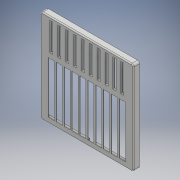
# Autodesk Inventor part: cover
Saved by Autodesk Inventor 2017 (Build 210142000, 142)
## iProperties
Created: 2017-08-24
Part Number: cover
Material: Generic
Document SubType Name: Modeling
Designer: erwin
Density: 1 g/cm^3
Appearance: Default
Author: erwin
Autodesk Inventor part; units mm, degrees
ref_plane "YZ Plane" through (0, 0, 0) normal (1, 0, 0) x (0, 1, 0)
ref_plane "XZ Plane" through (0, 0, 0) normal (0, 1, 0) x (-1, 0, 0)
ref_plane "XY Plane" through (0, 0, 0) normal (0, 0, 1) x (1, 0, 0)
sketch "Sketch1" plane through (0, 0, 0) normal (0, 1, 0) x (-1, 0, 0)
  line L0 (-45, 45) -> (45, 45)
  line L1 (45, 45) -> (45, -45)
  line L2 (45, -45) -> (-45, -45)
  line L3 (-45, -45) -> (-45, 45)
  line L4 (-45, 45) -> (45, -45) construction
  line L5 (45, 45) -> (-45, -45) construction
  line L6 (35.79, 42) -> (32.79, 42)
  line L7 (32.79, 42) -> (32.79, 15)
  line L8 (32.79, 15) -> (35.79, 15)
  line L9 (35.79, 15) -> (35.79, 42)
  line L10 (35.79, 42) -> (32.79, 15) construction
  line L11 (32.79, 42) -> (35.79, 15) construction
  line L12 (28.17, 42) -> (25.17, 42)
  line L13 (25.17, 42) -> (25.17, 15)
  line L14 (25.17, 15) -> (28.17, 15)
  line L15 (28.17, 15) -> (28.17, 42)
  line L16 (28.17, 42) -> (25.17, 15) construction
  line L17 (25.17, 42) -> (28.17, 15) construction
  line L18 (20.55, 42) -> (17.55, 42)
  line L19 (17.55, 42) -> (17.55, 15)
  line L20 (17.55, 15) -> (20.55, 15)
  line L21 (20.55, 15) -> (20.55, 42)
  line L22 (20.55, 42) -> (17.55, 15) construction
  line L23 (17.55, 42) -> (20.55, 15) construction
  line L24 (12.93, 42) -> (9.93, 42)
  line L25 (9.93, 42) -> (9.93, 15)
  line L26 (9.93, 15) -> (12.93, 15)
  line L27 (12.93, 15) -> (12.93, 42)
  line L28 (12.93, 42) -> (9.93, 15) construction
  line L29 (9.93, 42) -> (12.93, 15) construction
  line L30 (5.31, 42) -> (2.31, 42)
  line L31 (2.31, 42) -> (2.31, 15)
  line L32 (2.31, 15) -> (5.31, 15)
  line L33 (5.31, 15) -> (5.31, 42)
  line L34 (5.31, 42) -> (2.31, 15) construction
  line L35 (2.31, 42) -> (5.31, 15) construction
  line L36 (-2.31, 42) -> (-5.31, 42)
  line L37 (-5.31, 42) -> (-5.31, 15)
  line L38 (-5.31, 15) -> (-2.31, 15)
  line L39 (-2.31, 15) -> (-2.31, 42)
  line L40 (-2.31, 42) -> (-5.31, 15) construction
  line L41 (-5.31, 42) -> (-2.31, 15) construction
  line L42 (-9.93, 42) -> (-12.93, 42)
  line L43 (-12.93, 42) -> (-12.93, 15)
  line L44 (-12.93, 15) -> (-9.93, 15)
  line L45 (-9.93, 15) -> (-9.93, 42)
  line L46 (-9.93, 42) -> (-12.93, 15) construction
  line L47 (-12.93, 42) -> (-9.93, 15) construction
  line L48 (-17.55, 42) -> (-20.55, 42)
  line L49 (-20.55, 42) -> (-20.55, 15)
  line L50 (-20.55, 15) -> (-17.55, 15)
  line L51 (-17.55, 15) -> (-17.55, 42)
  line L52 (-17.55, 42) -> (-20.55, 15) construction
  line L53 (-20.55, 42) -> (-17.55, 15) construction
  line L54 (-25.17, 42) -> (-28.17, 42)
  line L55 (-28.17, 42) -> (-28.17, 15)
  line L56 (-28.17, 15) -> (-25.17, 15)
  line L57 (-25.17, 15) -> (-25.17, 42)
  line L58 (-25.17, 42) -> (-28.17, 15) construction
  line L59 (-28.17, 42) -> (-25.17, 15) construction
  line L60 (-32.79, 42) -> (-35.79, 42)
  line L61 (-35.79, 42) -> (-35.79, 15)
  line L62 (-35.79, 15) -> (-32.79, 15)
  line L63 (-32.79, 15) -> (-32.79, 42)
  line L64 (-32.79, 42) -> (-35.79, 15) construction
  line L65 (-35.79, 42) -> (-32.79, 15) construction
  line L66 (-35.79, 15) -> (35.79, 15) construction
  line L67 (35.79, 15) -> (35.79, 42) construction
  line L68 (35.79, 42) -> (-35.79, 42) construction
  line L69 (-35.79, 42) -> (-35.79, 15) construction
  line L70 (0, 42) -> (0, 45) construction
  line L71 (0, 42) -> (3, 42) construction
  line L72 (34.3728, 15) -> (34.3728, -45) construction
  line L73 (37.3728, 10) -> (31.3728, 10)
  line L74 (31.3728, 10) -> (31.3728, -40)
  line L75 (31.3728, -40) -> (37.3728, -40)
  line L76 (37.3728, -40) -> (37.3728, 10)
  line L77 (37.3728, 10) -> (31.3728, -40) construction
  line L78 (31.3728, 10) -> (37.3728, -40) construction
  line L79 (-52.62, 45) -> (37.38, -45) construction
  line L80 (23.7528, 10) -> (23.7528, -40)
  line L81 (23.7528, -40) -> (29.7528, -40)
  line L82 (29.7528, -40) -> (29.7528, 10)
  line L83 (29.7528, 10) -> (23.7528, -40) construction
  line L84 (23.7528, 10) -> (29.7528, -40) construction
  line L85 (29.7528, 10) -> (23.7528, 10)
  line L86 (-60.24, 45) -> (29.76, -45) construction
  line L87 (16.1328, 10) -> (16.1328, -40)
  line L88 (16.1328, -40) -> (22.1328, -40)
  line L89 (22.1328, -40) -> (22.1328, 10)
  line L90 (22.1328, 10) -> (16.1328, -40) construction
  line L91 (16.1328, 10) -> (22.1328, -40) construction
  line L92 (22.1328, 10) -> (16.1328, 10)
  line L93 (-67.86, 45) -> (22.14, -45) construction
  line L94 (8.5128, 10) -> (8.5128, -40)
  line L95 (8.5128, -40) -> (14.5128, -40)
  line L96 (14.5128, -40) -> (14.5128, 10)
  line L97 (14.5128, 10) -> (8.5128, -40) construction
  line L98 (8.5128, 10) -> (14.5128, -40) construction
  line L99 (14.5128, 10) -> (8.5128, 10)
  line L100 (-75.48, 45) -> (14.52, -45) construction
  line L101 (0.8928, 10) -> (0.8928, -40)
  line L102 (0.8928, -40) -> (6.8928, -40)
  line L103 (6.8928, -40) -> (6.8928, 10)
  line L104 (6.8928, 10) -> (0.8928, -40) construction
  line L105 (0.8928, 10) -> (6.8928, -40) construction
  line L106 (6.8928, 10) -> (0.8928, 10)
  line L107 (-83.1, 45) -> (6.9, -45) construction
  line L108 (-6.7272, 10) -> (-6.7272, -40)
  line L109 (-6.7272, -40) -> (-0.7272, -40)
  line L110 (-0.7272, -40) -> (-0.7272, 10)
  line L111 (-0.7272, 10) -> (-6.7272, -40) construction
  line L112 (-6.7272, 10) -> (-0.7272, -40) construction
  line L113 (-0.7272, 10) -> (-6.7272, 10)
  line L114 (-90.72, 45) -> (-0.72, -45) construction
  line L115 (-14.3472, 10) -> (-14.3472, -40)
  line L116 (-14.3472, -40) -> (-8.3472, -40)
  line L117 (-8.3472, -40) -> (-8.3472, 10)
  line L118 (-8.3472, 10) -> (-14.3472, -40) construction
  line L119 (-14.3472, 10) -> (-8.3472, -40) construction
  line L120 (-8.3472, 10) -> (-14.3472, 10)
  line L121 (-98.34, 45) -> (-8.34, -45) construction
  line L122 (-21.9672, 10) -> (-21.9672, -40)
  line L123 (-21.9672, -40) -> (-15.9672, -40)
  line L124 (-15.9672, -40) -> (-15.9672, 10)
  line L125 (-15.9672, 10) -> (-21.9672, -40) construction
  line L126 (-21.9672, 10) -> (-15.9672, -40) construction
  line L127 (-15.9672, 10) -> (-21.9672, 10)
  line L128 (-105.96, 45) -> (-15.96, -45) construction
  line L129 (-29.5872, 10) -> (-29.5872, -40)
  line L130 (-29.5872, -40) -> (-23.5872, -40)
  line L131 (-23.5872, -40) -> (-23.5872, 10)
  line L132 (-23.5872, 10) -> (-29.5872, -40) construction
  line L133 (-29.5872, 10) -> (-23.5872, -40) construction
  line L134 (-23.5872, 10) -> (-29.5872, 10)
  line L135 (-113.58, 45) -> (-23.58, -45) construction
  line L136 (-37.2072, 10) -> (-37.2072, -40)
  line L137 (-37.2072, -40) -> (-31.2072, -40)
  line L138 (-31.2072, -40) -> (-31.2072, 10)
  line L139 (-31.2072, 10) -> (-37.2072, -40) construction
  line L140 (-37.2072, 10) -> (-31.2072, -40) construction
  line L141 (-31.2072, 10) -> (-37.2072, 10)
  point P0 (0, 0)
  point P1 (34.29, 28.5)
  point P2 (26.67, 28.5)
  point P3 (19.05, 28.5)
  point P4 (11.43, 28.5)
  point P5 (3.81, 28.5)
  point P6 (-3.81, 28.5)
  point P7 (-11.43, 28.5)
  point P8 (-19.05, 28.5)
  point P9 (-26.67, 28.5)
  point P10 (-34.29, 28.5)
  point P11 (0, 45)
  point P12 (34.3728, -15)
  point P13 (26.7528, -15)
  point P14 (19.1328, -15)
  point P15 (11.5128, -15)
  point P16 (3.8928, -15)
  point P17 (-3.7272, -15)
  point P18 (-11.3472, -15)
  point P19 (-18.9672, -15)
  point P20 (-26.5872, -15)
  point P21 (-34.2072, -15)
  dimension "d0" = 90
  dimension "d1" = 90
  dimension "d2" = 3
  dimension "d3" = 27
  dimension "d6" = 7.62
  dimension "d11" = 3
  dimension "d12" = 90
  dimension "d13" = 6
  dimension "d14" = 50
  dimension "d17" = 7.62
  constraints: 284 end point, 45 midpoint, 8 parallel, 7 horizontal, 6 perpendicular, 2 collinear, 2 point on line, 1 vertical, 223 other
  measures "d0" distance of L1.end L2.end
  measures "d1" distance of L0.end L1.end
  measures "d2" distance of L8.end L7.end
  measures "d3" distance of L7.end L6.end
  measures "d6" distance of L6.start L12.start
  measures "d11" distance of L70.start L70.end
  measures "d12" angle of L71 L70
  measures "d13" distance of L75.end L74.end
  measures "d14" distance of L74.end L73.end
  measures "d17" distance of L0.start L79.start
extrude "Extrusion1" add sketch "Sketch1" along normal blind 0.5
sketch "Sketch2" plane through (0, 0.5, 0) normal (0, 1, 0) x (1, 0, 0)
  line L0 (31.2072, -10) -> (31.2072, 40)
  line L1 (31.2072, 40) -> (37.2072, 40)
  line L2 (37.2072, 40) -> (37.2072, -10)
  line L3 (37.2072, -10) -> (31.2072, -10)
  line L4 (23.5872, -10) -> (23.5872, 40)
  line L5 (23.5872, 40) -> (29.5872, 40)
  line L6 (29.5872, 40) -> (29.5872, -10)
  line L7 (29.5872, -10) -> (23.5872, -10)
  line L8 (15.9672, -10) -> (15.9672, 40)
  line L9 (15.9672, 40) -> (21.9672, 40)
  line L10 (21.9672, 40) -> (21.9672, -10)
  line L11 (21.9672, -10) -> (15.9672, -10)
  line L12 (8.3472, -10) -> (8.3472, 40)
  line L13 (8.3472, 40) -> (14.3472, 40)
  line L14 (14.3472, 40) -> (14.3472, -10)
  line L15 (14.3472, -10) -> (8.3472, -10)
  line L16 (0.7272, -10) -> (0.7272, 40)
  line L17 (0.7272, 40) -> (6.7272, 40)
  line L18 (6.7272, 40) -> (6.7272, -10)
  line L19 (6.7272, -10) -> (0.7272, -10)
  line L20 (-6.8928, -10) -> (-6.8928, 40)
  line L21 (-6.8928, 40) -> (-0.8928, 40)
  line L22 (-0.8928, 40) -> (-0.8928, -10)
  line L23 (-0.8928, -10) -> (-6.8928, -10)
  line L24 (-14.5128, -10) -> (-14.5128, 40)
  line L25 (-14.5128, 40) -> (-8.5128, 40)
  line L26 (-8.5128, 40) -> (-8.5128, -10)
  line L27 (-8.5128, -10) -> (-14.5128, -10)
  line L28 (-22.1328, -10) -> (-22.1328, 40)
  line L29 (-22.1328, 40) -> (-16.1328, 40)
  line L30 (-16.1328, 40) -> (-16.1328, -10)
  line L31 (-16.1328, -10) -> (-22.1328, -10)
  line L32 (-29.7528, -10) -> (-29.7528, 40)
  line L33 (-29.7528, 40) -> (-23.7528, 40)
  line L34 (-23.7528, 40) -> (-23.7528, -10)
  line L35 (-23.7528, -10) -> (-29.7528, -10)
  line L36 (-37.3728, -10) -> (-37.3728, 40)
  line L37 (-37.3728, 40) -> (-31.3728, 40)
  line L38 (-31.3728, 40) -> (-31.3728, -10)
  line L39 (-31.3728, -10) -> (-37.3728, -10)
  line L40 (32.79, -42) -> (32.79, -15) projected
  line L41 (32.79, -15) -> (35.79, -15) projected
  line L42 (35.79, -15) -> (35.79, -42) projected
  line L43 (35.79, -42) -> (32.79, -42) projected
  line L44 (25.17, -42) -> (25.17, -15) projected
  line L45 (25.17, -15) -> (28.17, -15) projected
  line L46 (28.17, -15) -> (28.17, -42) projected
  line L47 (28.17, -42) -> (25.17, -42) projected
  line L48 (17.55, -42) -> (17.55, -15) projected
  line L49 (17.55, -15) -> (20.55, -15) projected
  line L50 (20.55, -15) -> (20.55, -42) projected
  line L51 (20.55, -42) -> (17.55, -42) projected
  line L52 (9.93, -42) -> (9.93, -15) projected
  line L53 (9.93, -15) -> (12.93, -15) projected
  line L54 (12.93, -15) -> (12.93, -42) projected
  line L55 (12.93, -42) -> (9.93, -42) projected
  line L56 (2.31, -42) -> (2.31, -15) projected
  line L57 (2.31, -15) -> (5.31, -15) projected
  line L58 (5.31, -15) -> (5.31, -42) projected
  line L59 (5.31, -42) -> (2.31, -42) projected
  line L60 (-5.31, -42) -> (-5.31, -15) projected
  line L61 (-5.31, -15) -> (-2.31, -15) projected
  line L62 (-2.31, -15) -> (-2.31, -42) projected
  line L63 (-2.31, -42) -> (-5.31, -42) projected
  line L64 (-12.93, -42) -> (-12.93, -15) projected
  line L65 (-12.93, -15) -> (-9.93, -15) projected
  line L66 (-9.93, -15) -> (-9.93, -42) projected
  line L67 (-9.93, -42) -> (-12.93, -42) projected
  line L68 (-20.55, -42) -> (-20.55, -15) projected
  line L69 (-20.55, -15) -> (-17.55, -15) projected
  line L70 (-17.55, -15) -> (-17.55, -42) projected
  line L71 (-17.55, -42) -> (-20.55, -42) projected
  line L72 (-28.17, -42) -> (-28.17, -15) projected
  line L73 (-28.17, -15) -> (-25.17, -15) projected
  line L74 (-25.17, -15) -> (-25.17, -42) projected
  line L75 (-25.17, -42) -> (-28.17, -42) projected
  line L76 (-35.79, -42) -> (-35.79, -15) projected
  line L77 (-35.79, -15) -> (-32.79, -15) projected
  line L78 (-32.79, -15) -> (-32.79, -42) projected
  line L79 (-32.79, -42) -> (-35.79, -42) projected
  line L80 (-45, -45) -> (45, -45) projected
  line L81 (45, -45) -> (45, 45) projected
  line L82 (45, 45) -> (-45, 45) projected
  line L83 (-45, 45) -> (-45, -45) projected
  line L84 (37.2072, -10) -> (-37.3728, -10)
  line L85 (-37.3728, -10) -> (-37.3728, 40)
  line L86 (-37.3728, 40) -> (37.2072, 40)
  line L87 (37.2072, 40) -> (37.2072, -10)
  line L88 (-43.396, -12.9864) -> (42.604, -12.9864)
  line L89 (42.604, -12.9864) -> (42.604, 43.0136)
  line L90 (42.604, 43.0136) -> (-43.396, 43.0136)
  line L91 (-43.396, 43.0136) -> (-43.396, -12.9864)
  line L92 (-0.396, 43.0136) -> (-0.396, -106.8962) construction
  line L93 (-0.396, 43.0136) -> (149.5138, 43.0136) construction
  point P0 (0, 0)
  dimension "d24" = 56
  dimension "d25" = 86
  dimension "d26" = 90
  constraints: 100 end point, 4 perpendicular, 1 horizontal, 1 midpoint, 1 other
  measures "d24" distance of L88.end L89.end
  measures "d25" distance of L89.end L90.end
  measures "d26" angle of L92 L93
extrude "Extrusion2" add sketch "Sketch2" along normal blind 1.5 contours L83 L82 L81 L80
sketch "Sketch3" plane through (0, 2, 0) normal (0, 1, 0) x (1, 0, 0)
  line L0 (-43.396, -12.9864) -> (-43.396, 43.0136) projected
  line L1 (-43.396, 43.0136) -> (42.604, 43.0136) projected
  line L2 (42.604, 43.0136) -> (42.604, -12.9864) projected
  line L3 (42.604, -12.9864) -> (-43.396, -12.9864) projected
  line L4 (-35.79, -15) -> (-32.79, -15) projected
  line L5 (-32.79, -15) -> (-32.79, -42) projected
  line L6 (-32.79, -42) -> (-35.79, -42) projected
  line L7 (-35.79, -42) -> (-35.79, -15) projected
  line L8 (-28.17, -15) -> (-25.17, -15) projected
  line L9 (-25.17, -15) -> (-25.17, -42) projected
  line L10 (-25.17, -42) -> (-28.17, -42) projected
  line L11 (-28.17, -42) -> (-28.17, -15) projected
  line L12 (-20.55, -15) -> (-17.55, -15) projected
  line L13 (-17.55, -15) -> (-17.55, -42) projected
  line L14 (-17.55, -42) -> (-20.55, -42) projected
  line L15 (-20.55, -42) -> (-20.55, -15) projected
  line L16 (-12.93, -15) -> (-9.93, -15) projected
  line L17 (-9.93, -15) -> (-9.93, -42) projected
  line L18 (-9.93, -42) -> (-12.93, -42) projected
  line L19 (-12.93, -42) -> (-12.93, -15) projected
  line L20 (-5.31, -15) -> (-2.31, -15) projected
  line L21 (-2.31, -15) -> (-2.31, -42) projected
  line L22 (-2.31, -42) -> (-5.31, -42) projected
  line L23 (-5.31, -42) -> (-5.31, -15) projected
  line L24 (2.31, -15) -> (5.31, -15) projected
  line L25 (5.31, -15) -> (5.31, -42) projected
  line L26 (5.31, -42) -> (2.31, -42) projected
  line L27 (2.31, -42) -> (2.31, -15) projected
  line L28 (9.93, -15) -> (12.93, -15) projected
  line L29 (12.93, -15) -> (12.93, -42) projected
  line L30 (12.93, -42) -> (9.93, -42) projected
  line L31 (9.93, -42) -> (9.93, -15) projected
  line L32 (17.55, -15) -> (20.55, -15) projected
  line L33 (20.55, -15) -> (20.55, -42) projected
  line L34 (20.55, -42) -> (17.55, -42) projected
  line L35 (17.55, -42) -> (17.55, -15) projected
  line L36 (25.17, -15) -> (28.17, -15) projected
  line L37 (28.17, -15) -> (28.17, -42) projected
  line L38 (28.17, -42) -> (25.17, -42) projected
  line L39 (25.17, -42) -> (25.17, -15) projected
  line L40 (32.79, -15) -> (35.79, -15) projected
  line L41 (35.79, -15) -> (35.79, -42) projected
  line L42 (35.79, -42) -> (32.79, -42) projected
  line L43 (32.79, -42) -> (32.79, -15) projected
  line L44 (-45, -45) -> (45, -45) projected
  line L45 (45, -45) -> (45, 45) projected
  line L46 (45, 45) -> (-45, 45) projected
  line L47 (-45, 45) -> (-45, -45) projected
  line L48 (-43.5, -43.5) -> (43.5, -43.5)
  line L49 (43.5, -43.5) -> (43.5, 43.5)
  line L50 (43.5, 43.5) -> (-43.5, 43.5)
  line L51 (-43.5, 43.5) -> (-43.5, -43.5)
  point P0 (0, 0)
  dimension "d29" = 1.5
  constraints: 8 end point, 3 other
  measures "d29" distance between parallel lines of L47 L51
extrude "Extrusion3" add sketch "Sketch3" along normal blind 4 contours L47 L46 L45 L44
fillet "Fillet1" radius 2 8 edges at (45, 3, 45) (45, 3, -45) (-45, 3, 45) (-45, 3, -45) (43.5, 4, -43.5) (43.5, 4, 43.5) (-43.5, 4, -43.5) (-43.5, 4, 43.5)
fillet "Fillet2" radius 1 8 edges at (44.4142, 0, 44.4142) (0, 0, 45) (-44.4142, 0, 44.4142) (-45, 0, 0) (-44.4142, 0, -44.4142) (0, 0, -45) (44.4142, 0, -44.4142) (45, 0, 0)
sketch "Sketch4" plane through (43, 6, -45) normal (0, 0, -1) x (-1, 0, 0)
  line L0 (0, 0) -> (86, 0) projected
  line L1 (40, 2) -> (46, 2)
  line L2 (46, 2) -> (46, -2)
  line L3 (46, -2) -> (40, -2)
  line L4 (40, -2) -> (40, 2)
  line L5 (40, 2) -> (46, -2) construction
  line L6 (46, 2) -> (40, -2) construction
  point P0 (43, -6)
  point P1 (43, 0)
  dimension "d34" = 6
  dimension "d35" = 4
  constraints: 12 end point, 3 midpoint, 2 parallel, 1 horizontal, 1 perpendicular
  measures "d34" distance of L2.end L3.end
  measures "d35" distance of L1.end L2.end
extrude "Extrusion4" cut sketch "Sketch4" against normal blind 19.25
body "Solid1"
